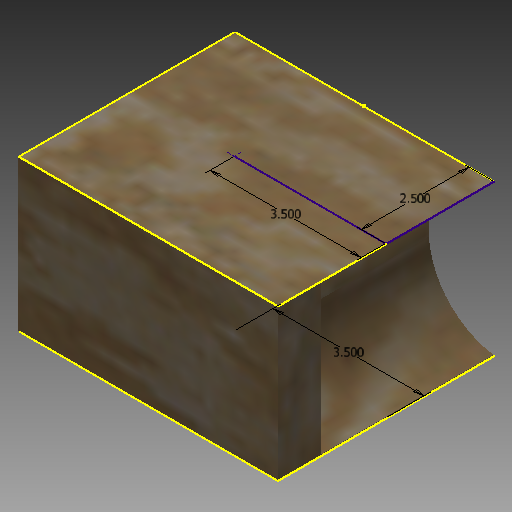
# Autodesk Inventor part: Holder
Saved by Autodesk Inventor 2017 (Build 210142000, 142)
## iProperties
Created: 2016-04-21
Part Number: Holder
Material: Generic
Document SubType Name: Modeling
Designer: Administrator
Density: 1 g/cm^3
Appearance: Plywood - Weathered
Author: Administrator
Autodesk Inventor part; units mm, degrees
ref_plane "YZ Plane" through (0, 0, 0) normal (1, 0, 0) x (0, 1, 0)
ref_plane "XZ Plane" through (0, 0, 0) normal (0, 1, 0) x (-1, 0, 0)
ref_plane "XY Plane" through (0, 0, 0) normal (0, 0, 1) x (1, 0, 0)
sketch "Sketch1" plane through (0, 0, 0) normal (0, 0, 1) x (1, 0, 0)
  line L0 (0, 0) -> (76.2, 0)
  line L1 (76.2, 0) -> (76.2, 88.9)
  line L2 (76.2, 88.9) -> (0, 88.9)
  line L3 (0, 88.9) -> (0, 0)
  dimension "d0" = 76.2
  dimension "d1" = 88.9
  constraints: 8 end point, 2 parallel, 1 horizontal, 1 perpendicular
  measures "d0" distance of L2.end L1.end
  measures "d1" distance of L1.end L0.end
extrude "Extrusion1" add sketch "Sketch1" along normal blind 127
sketch "Sketch3" plane through (0, 0, 0) normal (0, 0, -1) x (-1, 0, 0)
  circle A0 centre (-82.55, 44.45) radius 44.45
  dimension "d4" = 88.9
  constraints: 1 centre point
  measures "d4" diameter of A0
extrude "Extrusion2" cut sketch "Sketch3" against normal blind 101.6
sketch "Sketch4" plane through (0, 0, 0) normal (-1, 0, 0) x (0, 0, 1)
  line L0 (0, 0) -> (127, 0)
  line L1 (127, 0) -> (127, 88.9)
  line L2 (127, 88.9) -> (0, 88.9)
  line L3 (0, 88.9) -> (0, 0)
  constraints: 8 end point, 2 parallel, 1 horizontal, 1 perpendicular
extrude "Extrusion3" add sketch "Sketch4" along normal blind 76.2
sketch "Sketch5" plane through (76.2, 0, 0) normal (0, -1, 0) x (1, 0, 0)
  line L0 (-152.4, 0) -> (0, 0) projected
  line L1 (0, 0) -> (0, 127) projected
  line L2 (0, 127) -> (-152.4, 127) projected
  line L3 (-152.4, 0) -> (-152.4, 127) projected
  line L4 (0, 63.5) -> (-88.9, 63.5)
  point P0 (-76.2, 0)
  dimension "d9" = 88.9
  constraints: 2 end point, 1 coincident, 1 midpoint, 1 perpendicular
  measures "d9" distance of L4.start L4.end
sketch "Sketch6" plane through (76.2, 88.9, 127) normal (0, 1, 0) x (1, 0, 0)
  line L0 (0, 127) -> (-152.4, 127) projected
  line L1 (-152.4, 0) -> (-152.4, 127) projected
  line L2 (0, 0) -> (-152.4, 0) projected
  line L3 (0, 127) -> (0, 0) projected
  line L4 (0, 127) -> (0, 63.5)
  line L5 (0, 63.5) -> (-88.9, 63.5)
  point P0 (-76.2, 127)
  dimension "d10" = 63.5
  dimension "d11" = 88.9
  constraints: 4 end point, 1 coincident, 1 midpoint, 1 perpendicular
  measures "d10" distance of L0.start L4.end
  measures "d11" distance of L4.end L5.end
body "Solid1"
